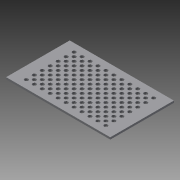
# Autodesk Inventor part: top
Saved by Autodesk Inventor 2013 SP1 (Build 170176100, 176)
## iProperties
Created: 2019-01-15
Part Number: top
Material: Типовые
Document SubType Name: Modeling
Designer: jhcjhguw
Density: 1 g/cm^3
Author: jhcjhguw
Autodesk Inventor part; units mm, degrees
ref_plane "YZ Plane" through (0, 0, 0) normal (1, 0, 0) x (0, 1, 0)
ref_plane "XZ Plane" through (0, 0, 0) normal (0, 1, 0) x (-1, 0, 0)
ref_plane "XY Plane" through (0, 0, 0) normal (0, 0, 1) x (1, 0, 0)
sketch "Эскиз1" plane through (0, 0, 0) normal (0, 0, 1) x (1, 0, 0)
  line L0 (0, 0) -> (104.8, 0)
  line L1 (104.8, 0) -> (104.8, 64)
  line L2 (104.8, 64) -> (0, 64)
  line L3 (0, 64) -> (0, 0)
  dimension "d0" = 104.8
  dimension "d1" = 64
  constraints: 8 end point, 2 parallel, 1 horizontal, 1 perpendicular
  measures "d0" distance of L2.end L1.end
  measures "d1" distance of L1.end L0.end
extrude "Выдавливание1" add sketch "Эскиз1" along normal blind 2
sketch "Эскиз2" plane through (0, 0, 2) normal (0, 0, 1) x (1, 0, 0)
  line L0 (0, 0) -> (104.8, 0) projected
  line L1 (0, 64) -> (0, 0) projected
  line L2 (10.6165, 8.375) -> (11.1835, 9.3571)
  line L3 (11.833, 9.7321) -> (12.967, 9.7321)
  line L4 (13.6165, 9.3571) -> (14.1835, 8.375)
  line L5 (14.1835, 7.625) -> (13.6165, 6.6429)
  line L6 (12.967, 6.2679) -> (11.833, 6.2679)
  line L7 (11.1835, 6.6429) -> (10.6165, 7.625)
  arc A0 (10.6165, 8.375) -> (10.6165, 7.625) centre (11.266, 8) ccw
  arc A1 (11.833, 9.7321) -> (11.1835, 9.3571) centre (11.833, 8.9821) ccw
  arc A2 (13.6165, 9.3571) -> (12.967, 9.7321) centre (12.967, 8.9821) ccw
  arc A3 (14.1835, 7.625) -> (14.1835, 8.375) centre (13.534, 8) ccw
  arc A4 (12.967, 6.2679) -> (13.6165, 6.6429) centre (12.967, 7.0179) ccw
  arc A5 (11.1835, 6.6429) -> (11.833, 6.2679) centre (11.833, 7.0179) ccw
  point P0 (12.4, 8)
  point P1 (10.4, 8)
  point P2 (11.4, 9.7321)
  point P3 (13.4, 9.7321)
  point P4 (14.4, 8)
  point P5 (13.4, 6.2679)
  point P6 (11.4, 6.2679)
  dimension "d4" = 2
  dimension "d5" = 0.75
  dimension "d6" = 12.4
  dimension "d7" = 8
  constraints: 12 end point, 12 point on circle, 12 point on line, 12 tangent, 6 centre point, 5 equal radius, 13 other
  measures "d4" distance of point (10.4, 8) point (12.4, 8)
  measures "d5" radius of A0
  measures "d6" distance from line of L1 point (12.4, 8)
  measures "d7" distance from line of L0 point (12.4, 8)
extrude "Выдавливание2" cut sketch "Эскиз2" against normal blind 2
pattern_linear "Прямоуг.массив1" count 7 spacing 8 along (0, 1, 0) count 11 spacing 8 along (1, 0, 0) of "Выдавливание2"
sketch "Эскиз3" plane through (0, 0, 2) normal (0, 0, 1) x (1, 0, 0)
  line L0 (0, 0) -> (104.8, 0) projected
  line L1 (0, 64) -> (0, 0) projected
  line L2 (18.1835, 11.625) -> (17.6165, 10.6429)
  line L3 (16.967, 10.2679) -> (15.833, 10.2679)
  line L4 (15.1835, 10.6429) -> (14.6165, 11.625)
  line L5 (14.6165, 12.375) -> (15.1835, 13.3571)
  line L6 (15.833, 13.7321) -> (16.967, 13.7321)
  line L7 (17.6165, 13.3571) -> (18.1835, 12.375)
  arc A0 (17.6165, 13.3571) -> (16.967, 13.7321) centre (16.967, 12.9821) ccw
  arc A1 (18.1835, 11.625) -> (18.1835, 12.375) centre (17.534, 12) ccw
  arc A2 (16.967, 10.2679) -> (17.6165, 10.6429) centre (16.967, 11.0179) ccw
  arc A3 (15.1835, 10.6429) -> (15.833, 10.2679) centre (15.833, 11.0179) ccw
  arc A4 (14.6165, 12.375) -> (14.6165, 11.625) centre (15.266, 12) ccw
  arc A5 (15.833, 13.7321) -> (15.1835, 13.3571) centre (15.833, 12.9821) ccw
  point P0 (16.4, 12)
  point P1 (18.4, 12)
  point P2 (17.4, 10.2679)
  point P3 (15.4, 10.2679)
  point P4 (14.4, 12)
  point P5 (15.4, 13.7321)
  point P6 (17.4, 13.7321)
  dimension "d16" = 2
  dimension "d17" = 16.4
  dimension "d18" = 12
  dimension "d19" = 0.75
  constraints: 12 end point, 12 point on circle, 12 point on line, 12 tangent, 6 centre point, 5 equal radius, 1 horizontal, 13 other
  measures "d16" distance of point (17.4, 10.268) point (15.4, 10.268)
  measures "d17" distance from line of L1 point (16.4, 12)
  measures "d18" distance from line of L0 point (16.4, 12)
  measures "d19" radius of A0
extrude "Выдавливание3" cut sketch "Эскиз3" against normal blind 2
pattern_linear "Прямоуг.массив2" count 6 spacing 8 along (0, 1, 0) count 10 spacing 8 along (1, 0, 0) of "Выдавливание3"
